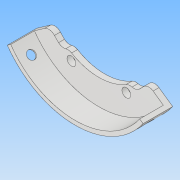
# Autodesk Inventor part: BearingMountBrace
Saved by Autodesk Inventor 2017.3 (Build 213256000, 256)
## iProperties
Created: 2019-06-27
Part Number: BearingMountBrace
Material: ABS Plastic
Document SubType Name: Modeling
Designer: Derek Wider
Density: 1.06 g/cm^3
Appearance: Smooth - White
Author: Derek Wider
Autodesk Inventor part; units mm, degrees
ref_plane "XZ Plane" through (0, 0, 0) normal (0, 1, 0) x (-1, 0, 0)
ref_plane "XY Plane" through (0, 0, 0) normal (0, 0, 1) x (1, 0, 0)
sketch "Sketch1" plane through (0, 0, 0) normal (0, 0, 1) x (1, 0, 0)
  arc A0 (-20.8065, -14.5688) -> (20.8065, -14.5688) centre (0, 0) ccw
  arc A1 (-29.129, -20.3964) -> (29.129, -20.3964) centre (0, 0) ccw
  line L0 (-29.129, -20.3964) -> (-20.8065, -14.5688)
  line L1 (29.129, -20.3964) -> (20.8065, -14.5688)
  line L2 (-20.8065, -14.5688) -> (20.8065, -14.5688) construction
  dimension "d0" = 50.8
  dimension "d2" = 71.12
  dimension "d3" = 110
  constraints: 6 end point, 4 point on circle, 2 centre point, 2 line through centre, 1 coincident, 1 horizontal
  measures "d0" diameter of A0
  measures "d2" diameter of A1
extrude "Extrusion1" add sketch "Sketch1" along normal blind 2.54
sketch "Sketch2" plane through (0, 0, 2.54) normal (0, 0, 1) x (1, 0, 0)
  arc A0 (-20.8065, -14.5688) -> (20.8065, -14.5688) centre (0, 0) ccw projected
  line L0 (-14.5688, -20.8065) -> (-13.112, -18.7258)
  line L1 (14.5688, -20.8065) -> (13.112, -18.7258)
  arc A1 (-13.112, -18.7258) -> (13.112, -18.7258) centre (0, 0) ccw
  line L2 (-14.5688, -20.8065) -> (14.5688, -20.8065) construction
  dimension "d6" = 2.54
  dimension "d13" = 70
  constraints: 6 end point, 4 point on circle, 2 line through centre, 1 centre point, 1 coincident, 1 horizontal
  measures "d6" distance of L0.start L0.end
extrude "Extrusion2" add sketch "Sketch2" against normal blind 2.54
sketch "Sketch3" plane through (0, 0, 2.54) normal (0, 0, 1) x (1, 0, 0)
  circle A0 centre (-11.7871, -22.6427) radius 1.905
  circle A1 centre (11.7871, -22.6427) radius 1.905
  line L0 (-11.7871, -22.6427) -> (11.7871, -22.6427) construction
  point P0 (0, 0)
  point P1 (0, -22.6427)
  dimension "d9" = 3.81
  dimension "d10" = 3.81
  dimension "d11" = 25.527
  dimension "d12" = 27.5
  constraints: 2 centre point, 2 end point, 1 horizontal, 1 midpoint, 1 vertical alignment
  measures "d9" diameter of A0
  measures "d10" diameter of A1
  measures "d11" distance of L0.start point (0, 0)
extrude "Extrusion3" cut sketch "Sketch3" against normal through all
sketch "Sketch4" plane through (0, 0, 2.54) normal (0, 0, 1) x (1, 0, 0)
  circle A0 centre (-11.7871, -22.6427) radius 1.905 projected
  circle A1 centre (11.7871, -22.6427) radius 1.905 projected
  arc A2 (-29.129, -20.3964) -> (29.129, -20.3964) centre (0, 0) ccw projected
  line L0 (29.129, -20.3964) -> (20.8065, -14.5688) projected
  arc A3 (14.5688, -20.8065) -> (20.8065, -14.5688) centre (0, 0) ccw projected
  line L1 (14.5688, -20.8065) -> (13.112, -18.7258) projected
  arc A4 (-13.112, -18.7258) -> (13.112, -18.7258) centre (0, 0) ccw projected
  line L2 (-13.112, -18.7258) -> (-14.5688, -20.8065) projected
  arc A5 (-20.8065, -14.5688) -> (-14.5688, -20.8065) centre (0, 0) ccw projected
  line L3 (-20.8065, -14.5688) -> (-29.129, -20.3964) projected
  line L4 (-20.8065, -14.5688) -> (-29.129, -20.3964) projected
  line L5 (29.129, -20.3964) -> (20.8065, -14.5688) projected
  arc A6 (-27.6726, -19.3766) -> (27.6726, -19.3766) centre (0, 0) ccw
  dimension "d17" = 67.564
  constraints: 2 point on circle, 2 point on line, 1 centre point, 1 coincident
  measures "d17" diameter of A6
extrude "Extrusion4" add sketch "Sketch4" along normal blind 10.16 contours L3 A6 L0 A2
ref_plane "Work Plane2" through (25.1447, -25.1447, 0) normal (0.7071068, -0.7071068, 0) x (0.7071068, 0.7071068, 0)
ref_plane "Work Plane1" through (0, 0, 2.54) normal (0.7071068, -0.7071068, 0) x (0, 0, -1)
ref_plane "Work Plane4" through (-25.1447, -25.1447, 0) normal (0.7071068, 0.7071068, 0) x (-0.7071068, 0.7071068, 0)
ref_plane "Work Plane3" through (0, 0, 2.54) normal (0.7071068, 0.7071068, 0) x (0, 0, -1)
sketch "Sketch5" plane through (-25.1447, -25.1447, 0) normal (0.7071068, 0.7071068, 0) x (-0.7071068, 0.7071068, 0)
  circle A0 centre (0, 7.62) radius 1.778
  line L0 (5.8662, 2.54) -> (5.8662, 12.7) projected
  point P0 (0, 0)
  point P1 (6.1749, 4.826)
  point P2 (5.8662, 7.62)
  dimension "d22" = 3.556
  constraints: 1 centre point, 1 horizontal alignment, 1 midpoint
  measures "d22" diameter of A0
extrude "Extrusion5" cut sketch "Sketch5" along normal blind 7.112
sketch "Sketch6" plane through (25.1447, -25.1447, 0) normal (0.7071068, -0.7071068, 0) x (0.7071068, 0.7071068, 0)
  circle A0 centre (0, 7.62) radius 1.778
  line L0 (5.8662, 2.54) -> (5.8662, 12.7) projected
  point P0 (0, 0)
  point P1 (6.1749, 4.826)
  point P2 (5.8662, 7.62)
  dimension "d25" = 3.556
  constraints: 1 centre point, 1 horizontal alignment, 1 midpoint
  measures "d25" diameter of A0
extrude "Extrusion6" cut sketch "Sketch6" against normal blind 7.112
fillet "Fillet1" radius 3.175 6 edges at (-20.8065, -14.5688, 1.27) (-14.5688, -20.8065, 1.27) (-13.112, -18.7258, 1.27) (13.112, -18.7258, 1.27) (14.5688, -20.8065, 1.27) (20.8065, -14.5688, 1.27)
chamfer "Chamfer1" distance 1.27 angle 45 2 edges at (-23.856, -26.3705, 7.6201) (23.856, -26.3705, 7.6201)
body "Solid1"
